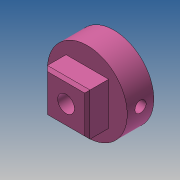
# Autodesk Inventor part: dado polea
Saved by Autodesk Inventor 2017 (Build 210142000, 142)
## iProperties
Part Number: dado polea
Material: Genérico
Document SubType Name: Modeling
Designer: Leo
Density: 1 g/cm^3
Appearance: Rosado
Description: Impresión 3d
Author: Leo
Autodesk Inventor part; units mm, degrees
ref_plane "YZ Plane" through (0, 0, 0) normal (1, 0, 0) x (0, 1, 0)
ref_plane "XZ Plane" through (0, 0, 0) normal (0, 1, 0) x (-1, 0, 0)
ref_plane "XY Plane" through (0, 0, 0) normal (0, 0, 1) x (1, 0, 0)
sketch "Boceto1" plane through (0, 0, 0) normal (0, 1, 0) x (-1, 0, 0)
  circle A0 centre (0, 0) radius 3.15
  circle A1 centre (0, 0) radius 15
  line L0 (-7.225, 3.7) -> (-10.925, 3.7)
  line L1 (-10.925, 3.7) -> (-10.925, -3.7)
  line L2 (-10.925, -3.7) -> (-7.225, -3.7)
  line L3 (-7.225, -3.7) -> (-7.225, 3.7)
  circle A2 centre (0, 0) radius 9.8003 construction
  line L4 (6.8168, -4.407) -> (0.4082, -8.107)
  line L5 (8.6668, -7.6113) -> (6.8168, -4.407)
  line L6 (2.2582, -11.3113) -> (8.6668, -7.6113)
  line L7 (0.4082, -8.107) -> (2.2582, -11.3113)
  line L8 (0.4082, 8.107) -> (6.8168, 4.407)
  line L9 (2.2582, 11.3113) -> (0.4082, 8.107)
  line L10 (8.6668, 7.6113) -> (2.2582, 11.3113)
  line L11 (6.8168, 4.407) -> (8.6668, 7.6113)
  point P0 (-7.225, 0)
  point P1 (-9.075, 3.7)
  point P2 (3.6125, -6.257)
  point P3 (1.3332, -9.7092)
  point P4 (3.6125, 6.257)
  point P5 (7.7418, 6.0092)
  dimension "d0" = 6.3
  dimension "tuerca" = 7.4
  dimension "d2" = 11.85
  dimension "d3" = 6.6503
  dimension "d4" = 3.7
  dimension "d18" = 360
  dimension "d26" = 30
  dimension "d27" = 4.075
  dimension "d28" = 4.075
  constraints: 24 end point, 2 centre point, 2 coincident, 2 midpoint, 2 parallel, 1 horizontal, 1 horizontal alignment, 1 perpendicular, 34 other
  measures "d0" diameter of A0
  measures "tuerca" distance of L0.end L1.end
  measures "d2" radial gap between concentric circles of A1 A0
  measures "d4" distance of L0.start L0.end
  measures "d26" diameter of A1
  measures "d27" distance edge to line of A0 L3
  measures "d28" distance edge to line of A1 L1
extrude "Extrusión1" add sketch "Boceto1" along normal blind 10 contours A1 | L5 L6 L7 L4 | L9 L10 L11 L8
sketch "Boceto2" plane through (7.225, 0, -3.7) normal (1, 0, 0) x (0, 0, -1)
  line L0 (0, 0) -> (-7.4, 0) projected
  line L1 (0, 0) -> (0, 10) construction
  line L2 (-7.4, 10) -> (0, 10) construction
  line L3 (-7.4, 0) -> (-7.4, 10) construction
  line L4 (-7.4, 0) -> (0, 10) construction
  circle A0 centre (-3.7, 5) radius 2.1
  line L5 (0, 2.6329) -> (-4.5603, 0)
  line L6 (-2.8397, 0) -> (-7.4, 2.6329)
  line L7 (-7.4, 2.6329) -> (-7.4, 0)
  line L8 (0, 2.6329) -> (0, 0)
  point P0 (-3.7, 0)
  dimension "d7" = 4.2
  dimension "d8" = 120
  dimension "d9" = 3.9
  constraints: 10 end point, 4 point on line, 1 centre point, 1 collinear, 1 equal length, 1 horizontal alignment, 1 midpoint
  measures "d7" diameter of A0
  measures "d8" angle of L5 L6
  measures "d9" distance from line of A0.centre L5
extrude "Extrusión2" cut sketch "Boceto2" along normal mid plane 16 contours A0
extrude "Extrusión3" add sketch "Boceto2" along normal up to next contours L0 L6 L5 L8 | L0 L5 L6 | L0 L7 L6 L5
sketch "Boceto3" plane through (0, 0, 0) normal (0, -1, 0) x (1, 0, 0)
  circle A0 centre (0, 0) radius 3.15 projected
  circle A1 centre (0, 0) radius 27.5
  line L0 (-8, 8) -> (8, 8)
  line L1 (8, 8) -> (8, -8)
  line L2 (8, -8) -> (-8, -8)
  line L3 (-8, -8) -> (-8, 8)
  point P0 (-8, 0)
  point P1 (0, 8)
  dimension "d32" = 16
  dimension "d33" = 55
  constraints: 8 end point, 2 midpoint, 2 parallel, 2 perpendicular, 1 centre point, 1 horizontal, 1 horizontal alignment, 1 vertical alignment
  measures "d32" distance of L0.end L1.end
  measures "d33" diameter of A1
extrude "Extrusión4" add sketch "Boceto3" along normal blind 8 contours L0 L1 L2 L3
chamfer "Chaflán1" distance 1 angle 45 2 edges at (9.075, 10, 3.7) (9.075, 10, -3.7)
chamfer "Chaflán3" distance 1 angle 45 4 edges at (0, -8, 8) (-8, -8, 0) (0, -8, -8) (8, -8, 0)
equation "\"d28\" = d27"
